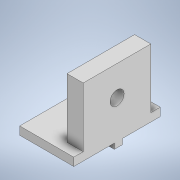
# Autodesk Inventor part: AlignmentJig
Saved by Autodesk Inventor 2021.1 (Build 251245010, 245A)
## iProperties
Created: 2021-09-28
Part Number: AlignmentJig
Material: Generic
Document SubType Name: Modeling
Designer: jloeb
Density: 1 g/cm^3
Appearance: Default
Author: jloeb
## iProperties of the stored document _3DPrint.ipt
Created: 2021-09-28
Part Number: _3DPrint
Material: Generic
Document SubType Name: Modeling
Designer: jloeb
Density: 1 g/cm^3
Appearance: Default
Author: jloeb
Autodesk Inventor part; units mm, degrees
ref_plane "YZ Plane" through (0, 0, 0) normal (1, 0, 0) x (0, 1, 0)
ref_plane "XZ Plane" through (0, 0, 0) normal (0, 1, 0) x (-1, 0, 0)
ref_plane "XY Plane" through (0, 0, 0) normal (0, 0, 1) x (1, 0, 0)
sketch "Sketch1" plane through (0, 0, 0) normal (1, 0, 0) x (0, 1, 0)
  line L0 (0, 0) -> (22, 0)
  line L1 (22, 0) -> (22, -25)
  line L2 (22, -25) -> (0, -25)
  line L3 (0, -25) -> (0, 0)
  circle A0 centre (11, -12.5) radius 2.6
  dimension "d0" = 22
  dimension "d1" = 25
  dimension "d2" = 5.2
  dimension "d3" = 11
  dimension "d4" = 12.5
  constraints: 8 end point, 2 parallel, 1 centre point, 1 horizontal, 1 perpendicular
  measures "d0" distance of L1.end L2.end
  measures "d1" distance of L0.end L1.end
  measures "d2" diameter of A0
  measures "d3" distance from line of L1 A0.centre
  measures "d4" distance from line of L0 A0.centre
extrude "Extrusion1" add sketch "Sketch1" along normal blind 6
sketch "Sketch2" plane through (6, 0, 0) normal (1, 0, 0) x (0, 0, -1)
  line L0 (-3.5, 0) -> (28.5, 0)
  line L1 (28.5, 0) -> (28.5, -3)
  line L2 (-3.5, -3) -> (-3.5, 0)
  line L3 (0, 22) -> (0, 0) projected
  line L4 (25, 0) -> (25, 22) projected
  line L5 (0, 0) -> (25, 0) projected
  line L6 (11.5, -3) -> (14.5, -3)
  line L7 (14.5, -3) -> (14.5, -5)
  line L8 (14.5, -5) -> (11.5, -5)
  line L9 (11.5, -5) -> (11.5, -3)
  line L10 (28.5, -3) -> (14.5, -3)
  line L11 (11.5, -3) -> (-3.5, -3)
  dimension "d8" = 3
  dimension "d9" = 3.5
  dimension "d10" = 3.5
  dimension "d13" = 3
  dimension "d14" = 2
  dimension "d15" = 11.5
  constraints: 18 end point, 5 parallel, 2 horizontal, 2 perpendicular, 1 collinear
  measures "d8" distance of L0.end L1.end
  measures "d9" distance between parallel lines of L3 L2
  measures "d10" distance between parallel lines of L4 L1
  measures "d13" distance of L7.end L8.end
  measures "d14" distance of L6.end L7.end
  measures "d15" distance between parallel lines of L3 L9
extrude "Extrusion2" add sketch "Sketch2" against normal blind 20
equation "\"d3\" = 0.5 * d0"
body "Solid1"
